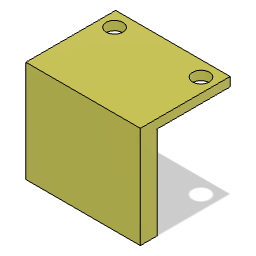
Device 3D Model (Autodesk Fusion 360 archive; units mm, degrees)
design "Accelerometer"
Autodesk Fusion 360 part; units mm, degrees
sketch "Sketch1" plane through (0, 0, 0) normal (0, 1, 0) x (1, 0, 0)
  line L0 (0, 0) -> (20.4, 0)
  line L1 (20.4, 0) -> (20.4, -16)
  line L2 (20.4, -16) -> (0, -16)
  line L3 (0, -16) -> (0, 0)
  dimension "d1" = 20.4
  dimension "d2" = 16
  constraint horizontal L0
  constraint vertical L1
  constraint horizontal L2
  constraint vertical L3
  constraint coincident L0.start L3.end
  measures "d1" distance of L0.start L0.end
  measures "d2" distance of L0.start L2.end
extrude "Extrude1" add sketch "Sketch1" along normal blind 1.6
sketch "Sketch2" plane through (0, 1.6, 0) normal (0, 1, 0) x (-1, 0, 0)
  line L0 (0, 16) -> (-20.4, 16)
  line L1 (-20.4, 16) -> (-20.4, 0)
  line L2 (-20.4, 0) -> (0, 0)
  line L3 (0, 0) -> (0, 16)
  line L4 (0, 1.2) -> (-20.4, 1.2)
  line L5 (0, 16) -> (-1, 16)
  line L6 (-20.4, 16) -> (-19.4, 16)
  line L7 (-1, 16) -> (-1, 0)
  line L8 (-19.4, 16) -> (-19.4, 0)
  circle A0 centre (-2.5, 2.7) radius 1.5
  circle A1 centre (-17.9, 2.7) radius 1.5
  dimension "d5" = 1.2
  dimension "d6" = 1
  dimension "d7" = 1
  dimension "d8" = 1.5
  dimension "d9" = 1.5
  constraint coincident L1 L4.end
  constraint perpendicular L1 L4
  constraint coincident L0.start L3.end
  constraint perpendicular L3 L5
  constraint coincident L0.end L1.start
  constraint perpendicular L1 L6
  constraint coincident L2 L7.end
  constraint perpendicular L2 L7
  constraint coincident L2 L8.end
  constraint perpendicular L2 L8
  constraint tangent L4 A0
  constraint tangent L7 A0
  constraint tangent L4 A1
  constraint tangent L8 A1
  measures "d5" distance of L2.end L4.start
  measures "d6" distance of L0.start L5.end
  measures "d7" distance of L0.end L6.end
  measures "d8" radius of A0
  measures "d9" radius of A1
extrude "Extrude2" cut sketch "Sketch2" against normal blind 15 contours A0 | A1
sketch "Sketch3" plane through (0, 0, 0) normal (0, -1, 0) x (1, 0, 0)
  circle A0 centre (2.5, 2.7) radius 1.5
  circle A1 centre (17.9, 2.7) radius 1.5
  line L0 (20.4, 16) -> (0, 16)
  line L1 (0, 16) -> (0, 0)
  line L2 (0, 0) -> (20.4, 0)
  line L3 (20.4, 0) -> (20.4, 16)
  line L4 (0, 16) -> (20.4, 16)
  line L5 (20.4, 16) -> (20.4, 13)
  line L6 (20.4, 13) -> (0, 13)
  line L7 (0, 13) -> (0, 16)
  dimension "d12" = 3
  constraint horizontal L4
  constraint vertical L5
  constraint horizontal L6
  constraint vertical L7
  constraint coincident L0.end L1.start
  measures "d12" distance of L0.end L6.end
extrude "Extrude3" add sketch "Sketch3" along normal blind 16.5 contours L0 L1 L3 L4 L5 L6 L7

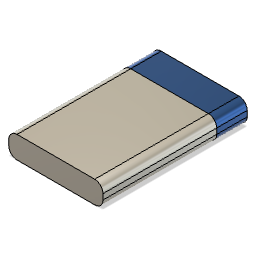
design "Battery"
Autodesk Fusion 360 part; units mm, degrees
sketch "Sketch1" plane through (0, 0, 0) normal (0, 1, 0) x (1, 0, 0)
  line L0 (0, 0) -> (34, 0)
  line L1 (34, 0) -> (34, -52)
  line L2 (34, -52) -> (0, -52)
  line L3 (0, -52) -> (0, 0)
  dimension "d1" = 34
  dimension "d2" = 52
  constraint horizontal L0
  constraint vertical L1
  constraint horizontal L2
  constraint vertical L3
  constraint coincident L0.start L3.end
  measures "d1" distance of L0.start L0.end
  measures "d2" distance of L0.start L2.end
extrude "Extrude1" add sketch "Sketch1" along normal blind 8 makes body 1
fillet "Fillet1" radius 3 4 edges at (34, 8, 26) (34, 0, 26) (0, 8, 26) (0, 0, 26) on bodies 1
ref_plane "WorkPlane1" through (17, 4, 11) normal (0, 0, -1) x (-1, 0, 0)
split "Split1" by plane through (17, 4, 11) normal (0, 0, -1) bodies 1 makes body 2 at (12.3333, 0, 3.6667)
copy_body "Body->Comp1" bodies 1 removing the originals makes body 3 in component "Component"
copy_body "Body->Comp2" bodies 2 removing the originals makes body 4 in component "Component'"
component "Component" placed x (1, 0, 0) y (0, 1, 0) z (0, 0, 1) at (0, 0, 0)
component "Component'" placed x (1, 0, 0) y (0, 1, 0) z (0, 0, 1) at (0, 0, 0)

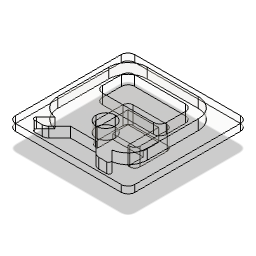
design "Logo"
Autodesk Fusion 360 part; units mm, degrees
sketch "Sketch1" plane through (0, 0, 0) normal (0, 1, 0) x (1, 0, 0)
  line L0 (0, 0) -> (30, 0)
  line L1 (30, 0) -> (30, -30)
  line L2 (30, -30) -> (0, -30)
  line L3 (0, -30) -> (0, 0)
  spline S0 degree 3 poles (5.625, 0) (2.5195, 0) (0, -2.5195) (0, -5.625) knots 0 0 0 0 1 1 1 1
  line L4 (0, -5.625) -> (0, -20.625)
  spline S1 degree 3 poles (0, -20.625) (0, -23.4375) (2.0625, -25.7637) (4.752, -26.1856) knots 0 0 0 0 1 1 1 1
  line L5 (4.752, -26.1856) -> (2.0566, -28.8809)
  spline S2 degree 3 poles (2.0566, -28.8809) (1.6465, -29.2911) (1.9395, -30) (2.5195, -30) knots 0 0 0 0 1 1 1 1
  line L6 (2.5195, -30) -> (4.8457, -30)
  spline S3 degree 3 poles (4.8457, -30) (5.3438, -30) (5.8184, -29.8008) (6.1699, -29.4493) knots 0 0 0 0 1 1 1 1
  line L7 (6.1699, -29.4493) -> (9.375, -26.25)
  line L8 (9.375, -26.25) -> (16.875, -26.25)
  line L9 (16.875, -26.25) -> (20.0742, -29.4493)
  spline S4 degree 3 poles (20.0742, -29.4493) (20.4258, -29.8008) (20.9004, -30) (21.3985, -30) knots 0 0 0 0 1 1 1 1
  line L10 (21.3985, -30) -> (23.7305, -30)
  spline S5 degree 3 poles (23.7305, -30) (24.3164, -30) (24.6094, -29.2911) (24.1934, -28.8809) knots 0 0 0 0 1 1 1 1
  line L11 (24.1934, -28.8809) -> (21.4981, -26.1856)
  spline S6 degree 3 poles (21.4981, -26.1856) (24.1934, -25.7696) (26.25, -23.4375) (26.25, -20.625) knots 0 0 0 0 1 1 1 1
  line L12 (26.25, -20.625) -> (26.25, -5.625)
  spline S7 degree 3 poles (26.25, -5.625) (26.25, -2.5195) (23.7305, 0) (20.625, 0) knots 0 0 0 0 1 1 1 1
  line L13 (20.625, 0) -> (5.625, 0)
  spline S8 degree 3 poles (3.75, -5.625) (3.75, -4.5879) (4.5879, -3.75) (5.625, -3.75) knots 0 0 0 0 1 1 1 1
  line L14 (5.625, -3.75) -> (20.625, -3.75)
  spline S9 degree 3 poles (20.625, -3.75) (21.6621, -3.75) (22.5, -4.5879) (22.5, -5.625) knots 0 0 0 0 1 1 1 1
  line L15 (22.5, -5.625) -> (22.5, -11.25)
  spline S10 degree 3 poles (22.5, -11.25) (22.5, -12.2871) (21.6621, -13.125) (20.625, -13.125) knots 0 0 0 0 1 1 1 1
  line L16 (20.625, -13.125) -> (5.625, -13.125)
  spline S11 degree 3 poles (5.625, -13.125) (4.5879, -13.125) (3.75, -12.2871) (3.75, -11.25) knots 0 0 0 0 1 1 1 1
  line L17 (3.75, -11.25) -> (3.75, -5.625)
  spline S12 degree 3 poles (13.125, -22.5) (11.5723, -22.5) (10.3125, -21.2403) (10.3125, -19.6875) knots 0 0 0 0 1 1 1 1
  spline S13 degree 3 poles (10.3125, -19.6875) (10.3125, -18.1348) (11.5723, -16.875) (13.125, -16.875) knots 0 0 0 0 1 1 1 1
  spline S14 degree 3 poles (13.125, -16.875) (14.6778, -16.875) (15.9375, -18.1348) (15.9375, -19.6875) knots 0 0 0 0 1 1 1 1
  spline S15 degree 3 poles (15.9375, -19.6875) (15.9375, -21.2403) (14.6778, -22.5) (13.125, -22.5) knots 0 0 0 0 1 1 1 1
  dimension "d1" = 30
  dimension "d2" = 30
  constraint horizontal L0
  constraint vertical L1
  constraint horizontal L2
  constraint vertical L3
  constraint coincident L0.start L3.end
  measures "d1" distance of L0.start L0.end
  measures "d2" distance of L0.start L2.end
extrude "Extrude1" add sketch "Sketch1" along normal blind 3 contours L0 L2 L3 S0 L4 S1 L5 S2 L6 S3 L7 L8 L9 S4 L10 S5 L11 S6 L12 S7 L13 makes body 1
sketch "Sketch2" plane through (0, 0, 0) normal (0, -1, 0) x (1, 0, 0)
  spline S0 degree 3 poles (5.625, 13.125) (4.5879, 13.125) (3.75, 12.2871) (3.75, 11.25) knots 0 0 0 0 1 1 1 1
  line L0 (5.625, 13.125) -> (20.625, 13.125)
  spline S1 degree 3 poles (22.5, 11.25) (22.5, 12.2871) (21.6621, 13.125) (20.625, 13.125) knots 0 0 0 0 1 1 1 1
  line L1 (22.5, 11.25) -> (22.5, 5.625)
  spline S2 degree 3 poles (20.625, 3.75) (21.6621, 3.75) (22.5, 4.5879) (22.5, 5.625) knots 0 0 0 0 1 1 1 1
  line L2 (20.625, 3.75) -> (5.625, 3.75)
  spline S3 degree 3 poles (3.75, 5.625) (3.75, 4.5879) (4.5879, 3.75) (5.625, 3.75) knots 0 0 0 0 1 1 1 1
  line L3 (3.75, 5.625) -> (3.75, 11.25)
  spline S4 degree 3 poles (13.125, 16.875) (14.6778, 16.875) (15.9375, 18.1348) (15.9375, 19.6875) knots 0 0 0 0 1 1 1 1
  spline S5 degree 3 poles (10.3125, 19.6875) (10.3125, 18.1348) (11.5723, 16.875) (13.125, 16.875) knots 0 0 0 0 1 1 1 1
  spline S6 degree 3 poles (13.125, 22.5) (11.5723, 22.5) (10.3125, 21.2403) (10.3125, 19.6875) knots 0 0 0 0 1 1 1 1
  spline S7 degree 3 poles (15.9375, 19.6875) (15.9375, 21.2403) (14.6778, 22.5) (13.125, 22.5) knots 0 0 0 0 1 1 1 1
  spline S8 degree 3 poles (23.7383, 30) (24.319, 29.9938) (24.6076, 29.2892) (24.1934, 28.8809) knots 0.004427 0.004427 0.004427 0.004427 1 1 1 1
  line L4 (23.7383, 30) -> (21.386, 30)
  spline S9 degree 3 poles (20.0742, 29.4493) (20.4229, 29.7979) (20.8925, 29.9967) (21.386, 30) knots 0 0 0 0 0.991654 0.991654 0.991654 0.991654
  line L5 (20.0742, 29.4493) -> (16.875, 26.25)
  line L6 (16.875, 26.25) -> (9.375, 26.25)
  line L7 (9.375, 26.25) -> (6.1699, 29.4493)
  spline S10 degree 3 poles (4.8582, 30) (5.3517, 29.9967) (5.8213, 29.7979) (6.1699, 29.4493) knots 0.008346 0.008346 0.008346 0.008346 1 1 1 1
  line L8 (4.8582, 30) -> (2.5118, 30)
  spline S11 degree 3 poles (2.0566, 28.8809) (1.6483, 29.2892) (1.9369, 29.9938) (2.5118, 30) knots 0 0 0 0 0.995573 0.995573 0.995573 0.995573
  line L9 (2.0566, 28.8809) -> (4.752, 26.1856)
  spline S12 degree 3 poles (0, 20.625) (0, 23.4375) (2.0625, 25.7637) (4.752, 26.1856) knots 0 0 0 0 1 1 1 1
  line L10 (0, 20.625) -> (0, 5.625)
  spline S13 degree 3 poles (5.625, 0) (2.5195, 0) (0, 2.5195) (0, 5.625) knots 0 0 0 0 1 1 1 1
  line L11 (5.625, 0) -> (20.625, 0)
  spline S14 degree 3 poles (26.25, 5.625) (26.25, 2.5195) (23.7305, 0) (20.625, 0) knots 0 0 0 0 1 1 1 1
  line L12 (26.25, 5.625) -> (26.25, 20.625)
  spline S15 degree 3 poles (21.4981, 26.1856) (24.1934, 25.7696) (26.25, 23.4375) (26.25, 20.625) knots 0 0 0 0 1 1 1 1
  line L13 (21.4981, 26.1856) -> (24.1934, 28.8809)
  circle A0 centre (13.125, 19.6875) radius 4.1368
extrude "Extrude2" add sketch "Sketch2" along normal blind 1 contours S4 S5 S6 S7 | S8 L4 S9 L5 L6 L7 S10 L8 S11 L9 S12 L10 S13 L11 S14 L12 S15 L13 | A0 bodies 1
sketch "Sketch3" plane through (0, -1, 0) normal (0, -1, 0) x (1, 0, 0)
  spline S0 degree 3 poles (22.5, 5.625) (22.5, 4.5879) (21.6621, 3.75) (20.625, 3.75) knots -1 -1 -1 -1 0 0 0 0
  line L0 (20.625, 3.75) -> (5.625, 3.75)
  spline S1 degree 3 poles (5.625, 3.75) (4.5879, 3.75) (3.75, 4.5879) (3.75, 5.625) knots -1 -1 -1 -1 0 0 0 0
  line L1 (3.75, 5.625) -> (3.75, 11.25)
  spline S2 degree 3 poles (3.75, 11.25) (3.75, 12.2871) (4.5879, 13.125) (5.625, 13.125) knots -1 -1 -1 -1 0 0 0 0
  line L2 (5.625, 13.125) -> (20.625, 13.125)
  spline S3 degree 3 poles (20.625, 13.125) (21.6621, 13.125) (22.5, 12.2871) (22.5, 11.25) knots -1 -1 -1 -1 0 0 0 0
  line L3 (22.5, 11.25) -> (22.5, 5.625)
  line L4 (26.25, 5.625) -> (26.25, 20.625)
  spline S4 degree 3 poles (26.25, 20.625) (26.25, 23.4375) (24.1934, 25.7696) (21.4981, 26.1856) knots -1 -1 -1 -1 0 0 0 0
  line L5 (21.4981, 26.1856) -> (24.1934, 28.8809)
  spline S5 degree 3 poles (24.1934, 28.8809) (24.6076, 29.2892) (24.319, 29.9938) (23.7383, 30) knots -1 -1 -1 -1 -0.004427 -0.004427 -0.004427 -0.004427
  line L6 (23.7383, 30) -> (21.386, 30)
  spline S6 degree 3 poles (21.386, 30) (20.8925, 29.9967) (20.4229, 29.7979) (20.0742, 29.4493) knots -0.991654 -0.991654 -0.991654 -0.991654 0 0 0 0
  line L7 (20.0742, 29.4493) -> (16.875, 26.25)
  line L8 (16.875, 26.25) -> (9.375, 26.25)
  line L9 (9.375, 26.25) -> (6.1699, 29.4493)
  spline S7 degree 3 poles (6.1699, 29.4493) (5.8213, 29.7979) (5.3517, 29.9967) (4.8582, 30) knots -1 -1 -1 -1 -0.008346 -0.008346 -0.008346 -0.008346
  line L10 (4.8582, 30) -> (2.5118, 30)
  spline S8 degree 3 poles (2.5118, 30) (1.9369, 29.9938) (1.6483, 29.2892) (2.0566, 28.8809) knots -0.995573 -0.995573 -0.995573 -0.995573 0 0 0 0
  line L11 (2.0566, 28.8809) -> (4.752, 26.1856)
  spline S9 degree 3 poles (4.752, 26.1856) (2.0625, 25.7637) (0, 23.4375) (0, 20.625) knots -1 -1 -1 -1 0 0 0 0
  line L12 (0, 20.625) -> (0, 5.625)
  spline S10 degree 3 poles (0, 5.625) (0, 2.5195) (2.5195, 0) (5.625, 0) knots -1 -1 -1 -1 0 0 0 0
  line L13 (5.625, 0) -> (20.625, 0)
  spline S11 degree 3 poles (20.625, 0) (23.7305, 0) (26.25, 2.5195) (26.25, 5.625) knots -1 -1 -1 -1 0 0 0 0
  line L14 (23.5046, 3.0171) -> (3, 3.0171)
  line L15 (3, 3.0171) -> (3, 15)
  line L16 (3, 15) -> (23.5046, 15)
  line L17 (23.5046, 15) -> (23.5046, 3.0171)
  constraint horizontal L14
  constraint vertical L15
  constraint horizontal L16
  constraint vertical L17
extrude "Extrude3" add sketch "Sketch3" against normal blind 1 contours S0 L0 S1 L1 S2 L2 S3 L3 bodies 1
sketch "Sketch4" plane through (0, -1, 0) normal (0, -1, 0) x (1, 0, 0)
  line L0 (26.25, 5.625) -> (26.25, 20.625)
  spline S0 degree 3 poles (26.25, 20.625) (26.25, 23.4375) (24.1934, 25.7696) (21.4981, 26.1856) knots -1 -1 -1 -1 0 0 0 0
  line L1 (21.4981, 26.1856) -> (24.1934, 28.8809)
  spline S1 degree 3 poles (24.1934, 28.8809) (24.6076, 29.2892) (24.319, 29.9938) (23.7383, 30) knots -1 -1 -1 -1 -0.004427 -0.004427 -0.004427 -0.004427
  line L2 (23.7383, 30) -> (21.386, 30)
  spline S2 degree 3 poles (21.386, 30) (20.8925, 29.9967) (20.4229, 29.7979) (20.0742, 29.4493) knots -0.991654 -0.991654 -0.991654 -0.991654 0 0 0 0
  line L3 (20.0742, 29.4493) -> (16.875, 26.25)
  line L4 (16.875, 26.25) -> (9.375, 26.25)
  line L5 (9.375, 26.25) -> (6.1699, 29.4493)
  spline S3 degree 3 poles (6.1699, 29.4493) (5.8213, 29.7979) (5.3517, 29.9967) (4.8582, 30) knots -1 -1 -1 -1 -0.008346 -0.008346 -0.008346 -0.008346
  line L6 (4.8582, 30) -> (2.5118, 30)
  spline S4 degree 3 poles (2.5118, 30) (1.9369, 29.9938) (1.6483, 29.2892) (2.0566, 28.8809) knots -0.995573 -0.995573 -0.995573 -0.995573 0 0 0 0
  line L7 (2.0566, 28.8809) -> (4.752, 26.1856)
  spline S5 degree 3 poles (4.752, 26.1856) (2.0625, 25.7637) (0, 23.4375) (0, 20.625) knots -1 -1 -1 -1 0 0 0 0
  line L8 (0, 20.625) -> (0, 5.625)
  spline S6 degree 3 poles (0, 5.625) (0, 2.5195) (2.5195, 0) (5.625, 0) knots -1 -1 -1 -1 0 0 0 0
  line L9 (5.625, 0) -> (20.625, 0)
  spline S7 degree 3 poles (20.625, 0) (23.7305, 0) (26.25, 2.5195) (26.25, 5.625) knots -1 -1 -1 -1 0 0 0 0
  line L10 (10.625, 15.625) -> (15.625, 15.625)
  line L11 (15.625, 15.625) -> (15.625, 10.625)
  line L12 (15.625, 10.625) -> (10.625, 10.625)
  line L13 (10.625, 10.625) -> (10.625, 15.625)
  line L14 (10.625, 15.625) -> (15.625, 10.625) construction
  line L15 (15.625, 15.625) -> (10.625, 10.625) construction
  line L16 (8.625, 17.625) -> (17.625, 17.625)
  line L17 (17.625, 17.625) -> (17.625, 8.625)
  line L18 (17.625, 8.625) -> (8.625, 8.625)
  line L19 (8.625, 8.625) -> (8.625, 17.625)
  line L20 (6.625, 19.625) -> (19.625, 19.625)
  line L21 (19.625, 19.625) -> (19.625, 6.625)
  line L22 (19.625, 6.625) -> (6.625, 6.625)
  line L23 (6.625, 6.625) -> (6.625, 19.625)
  line L24 (17.625, 17.625) -> (19.625, 17.625)
  line L25 (19.625, 17.625) -> (19.625, 6.625)
  line L26 (19.625, 6.625) -> (17.625, 6.625)
  line L27 (17.625, 8.625) -> (17.625, 17.625)
  line L28 (8.625, 17.625) -> (6.625, 17.625)
  line L29 (6.625, 17.625) -> (6.625, 6.625)
  line L30 (6.625, 6.625) -> (8.625, 6.625)
  line L31 (8.625, 8.625) -> (8.625, 17.625)
  dimension "d9" = 5
  dimension "d10" = 5
  dimension "d11" = -2
  dimension "d12" = -4
  constraint horizontal L10
  constraint perpendicular L10 L11
  constraint parallel L10 L12
  constraint parallel L11 L13
  constraint horizontal L24
  constraint vertical L25
  constraint horizontal L26
  constraint vertical L27
  constraint horizontal L28
  constraint vertical L29
  constraint horizontal L30
  constraint vertical L31
  measures "d9" distance of L11.end L12.end
  measures "d10" distance of L10.end L11.end
extrude "Extrude4" add sketch "Sketch4" along normal blind 2.8 contours L17 L18 L19 L21 L22 L23 L24 L25 L26 L27 L28 L29 L30 L31 bodies 1
sketch "Sketch5" plane through (0, -3.8, 0) normal (0, -1, 0) x (1, 0, 0)
  line L0 (17.625, 8.625) -> (8.625, 8.625)
  line L1 (8.625, 8.625) -> (8.625, 17.625)
  line L2 (8.625, 17.625) -> (6.625, 17.625)
  line L3 (6.625, 17.625) -> (6.625, 6.625)
  line L4 (6.625, 6.625) -> (19.625, 6.625)
  line L5 (19.625, 6.625) -> (19.625, 17.625)
  line L6 (19.625, 17.625) -> (17.625, 17.625)
  line L7 (17.625, 17.625) -> (17.625, 8.625)
  line L8 (19.625, 6.625) -> (6.625, 6.625)
  line L9 (6.625, 6.625) -> (6.625, 17.625)
  line L10 (6.625, 17.625) -> (19.625, 17.625)
  line L11 (19.625, 17.625) -> (19.625, 6.625)
  constraint horizontal L8
  constraint vertical L9
  constraint horizontal L10
  constraint vertical L11
  constraint coincident L2.end L3.start
  constraint coincident L4.end L5.start
extrude "Extrude5" add sketch "Sketch5" along normal blind 1.5 bodies 1
fillet "Fillet1" radius 1.5 4 edges at (19.625, -3.15, 6.625) (19.625, -3.15, 17.625) (6.625, -3.15, 17.625) (6.625, -3.15, 6.625) on bodies 1
extrude "Extrude6" cut 1 faces at (11.4584, -5.3, 13.9584) along direction (0, 1, 0) blind 1.5 on bodies 1 bodies 1
extrude "Extrude7" add 1 faces at (7.9584, -3.8, 14.125) along direction (0, -1, 0) blind 1 on bodies 1 bodies 1
sketch "Sketch6" plane through (0, -4.8, 0) normal (0, -1, 0) x (1, 0, 0)
  line L0 (17.625, 17.625) -> (17.625, 8.625)
  line L1 (17.625, 8.625) -> (8.625, 8.625)
  line L2 (8.625, 8.625) -> (8.625, 17.625)
  line L3 (8.625, 17.625) -> (8.125, 17.625)
  arc A0 (8.125, 17.625) -> (6.625, 16.125) centre (8.125, 16.125) ccw
  line L4 (6.625, 16.125) -> (6.625, 8.125)
  arc A1 (6.625, 8.125) -> (8.125, 6.625) centre (8.125, 8.125) ccw
  line L5 (8.125, 6.625) -> (18.125, 6.625)
  arc A2 (18.125, 6.625) -> (19.625, 8.125) centre (18.125, 8.125) ccw
  line L6 (19.625, 8.125) -> (19.625, 16.125)
  arc A3 (19.625, 16.125) -> (18.125, 17.625) centre (18.125, 16.125) ccw
  line L7 (18.125, 17.625) -> (17.625, 17.625)
  line L8 (17.625, 8.625) -> (8.625, 8.625)
  line L9 (8.625, 8.625) -> (8.625, 13.125)
  line L10 (8.625, 13.125) -> (17.625, 13.125)
  line L11 (17.625, 13.125) -> (17.625, 8.625)
  constraint horizontal L8
  constraint vertical L9
  constraint horizontal L10
  constraint vertical L11
  constraint midpoint L2 L9.end
  constraint coincident L0.end L1.start
extrude "Extrude8" add sketch "Sketch6" along normal blind 1 bodies 1
extrude "Extrude9" add 1 faces at (14.625, -5.8, 8.7917) along direction (0, -1, 0) blind 0.5 on bodies 1 bodies 1
sketch "Sketch7" plane through (0, -1, 0) normal (0, -1, 0) x (1, 0, 0)
  line L0 (17.625, 8.625) -> (17.625, 17.625)
  line L1 (17.625, 17.625) -> (18.125, 17.625)
  arc A0 (19.625, 16.125) -> (18.125, 17.625) centre (18.125, 16.125) ccw
  line L2 (19.625, 16.125) -> (19.625, 8.125)
  arc A1 (18.125, 6.625) -> (19.625, 8.125) centre (18.125, 8.125) ccw
  line L3 (18.125, 6.625) -> (8.125, 6.625)
  arc A2 (6.625, 8.125) -> (8.125, 6.625) centre (8.125, 8.125) ccw
  line L4 (6.625, 8.125) -> (6.625, 16.125)
  arc A3 (8.125, 17.625) -> (6.625, 16.125) centre (8.125, 16.125) ccw
  line L5 (8.125, 17.625) -> (8.625, 17.625)
  line L6 (8.625, 17.625) -> (8.625, 8.625)
  line L7 (8.625, 8.625) -> (17.625, 8.625)
  line L8 (26.25, 5.625) -> (26.25, 20.625)
  spline S0 degree 3 poles (26.25, 20.625) (26.25, 23.4375) (24.1934, 25.7696) (21.4981, 26.1856) knots -1 -1 -1 -1 0 0 0 0
  line L9 (21.4981, 26.1856) -> (24.1934, 28.8809)
  spline S1 degree 3 poles (24.1934, 28.8809) (24.6076, 29.2892) (24.319, 29.9938) (23.7383, 30) knots -1 -1 -1 -1 -0.004427 -0.004427 -0.004427 -0.004427
  line L10 (23.7383, 30) -> (21.386, 30)
  spline S2 degree 3 poles (21.386, 30) (20.8925, 29.9967) (20.4229, 29.7979) (20.0742, 29.4493) knots -0.991654 -0.991654 -0.991654 -0.991654 0 0 0 0
  line L11 (20.0742, 29.4493) -> (16.875, 26.25)
  line L12 (16.875, 26.25) -> (9.375, 26.25)
  line L13 (9.375, 26.25) -> (6.1699, 29.4493)
  spline S3 degree 3 poles (6.1699, 29.4493) (5.8213, 29.7979) (5.3517, 29.9967) (4.8582, 30) knots -1 -1 -1 -1 -0.008346 -0.008346 -0.008346 -0.008346
  line L14 (4.8582, 30) -> (2.5118, 30)
  spline S4 degree 3 poles (2.5118, 30) (1.9369, 29.9938) (1.6483, 29.2892) (2.0566, 28.8809) knots -0.995573 -0.995573 -0.995573 -0.995573 0 0 0 0
  line L15 (2.0566, 28.8809) -> (4.752, 26.1856)
  spline S5 degree 3 poles (4.752, 26.1856) (2.0625, 25.7637) (0, 23.4375) (0, 20.625) knots -1 -1 -1 -1 0 0 0 0
  line L16 (0, 20.625) -> (0, 5.625)
  spline S6 degree 3 poles (0, 5.625) (0, 2.5195) (2.5195, 0) (5.625, 0) knots -1 -1 -1 -1 0 0 0 0
  line L17 (5.625, 0) -> (20.625, 0)
  spline S7 degree 3 poles (20.625, 0) (23.7305, 0) (26.25, 2.5195) (26.25, 5.625) knots -1 -1 -1 -1 0 0 0 0
  line L18 (13.125, 0) -> (13.125, 26.25)
  line L19 (26.25, 13.125) -> (0, 13.125)
  line L20 (30.625, 30.625) -> (-4.375, 30.625)
  line L21 (-4.375, 30.625) -> (-4.375, -4.375)
  line L22 (-4.375, -4.375) -> (30.625, -4.375)
  line L23 (30.625, -4.375) -> (30.625, 30.625)
  line L24 (30.625, 30.625) -> (-4.375, -4.375) construction
  line L25 (-4.375, 30.625) -> (30.625, -4.375) construction
  point P0 (13.125, 13.125)
  dimension "d27" = 35
  dimension "d28" = 35
  constraint midpoint L17 L18.start
  constraint midpoint L12 L18.end
  constraint midpoint L8 L19.start
  constraint midpoint L16 L19.end
  constraint horizontal L20
  constraint perpendicular L20 L21
  constraint parallel L20 L22
  constraint parallel L21 L23
  constraint coincident L24 P0
  constraint coincident L25 P0
  constraint midpoint L19 P0
  measures "d27" distance of L21.end L22.end
  measures "d28" distance of L20.end L21.end
extrude "Extrude10" add sketch "Sketch7" against normal blind 1 bodies 1
split "Split1" by plane through (0, -1, 0) normal (0, -1, 0) bodies 1 makes body 2 at (14.625, -6.3, 8.7917)
move_body "Move1" bodies 2 to x (1, 0, 0) y (0, 1, 0) z (0, 0, 1) at (0, -1, 0)
extrude "Extrude11" add 3 faces at (13.125, -1, -2.9167) (13.125, -1, 20.5) (18.2917, -1, 14.125) along direction (0, -1, 0) blind 1 on bodies 1 bodies 1 2
fillet "Fillet2" radius 2 4 edges at (-4.375, -1, 30.625) (30.625, -1, 30.625) (30.625, -1, -4.375) (-4.375, -1, -4.375) on bodies 1
named bodies: "Logo", "Logo (1)"

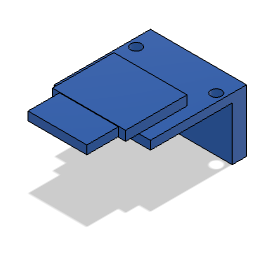
design "SDCard"
Autodesk Fusion 360 part; units mm, degrees
sketch "Sketch1" plane through (0, 0, 0) normal (0, 1, 0) x (1, 0, 0)
  line L0 (0, 0) -> (18, 0)
  line L1 (18, 0) -> (18, -18)
  line L2 (18, -18) -> (0, -18)
  line L3 (0, -18) -> (0, 0)
  dimension "d1" = 18
  dimension "d2" = 18
  constraint horizontal L0
  constraint vertical L1
  constraint horizontal L2
  constraint vertical L3
  constraint coincident L0.start L3.end
  measures "d1" distance of L0.start L0.end
  measures "d2" distance of L0.start L2.end
extrude "Extrude1" add sketch "Sketch1" along normal blind 1.6
sketch "Sketch2" plane through (0, 1.6, 0) normal (0, 1, 0) x (-1, 0, 0)
  line L0 (0, 18) -> (-18, 18)
  line L1 (-18, 18) -> (-18, 0)
  line L2 (-18, 0) -> (0, 0)
  line L3 (0, 0) -> (0, 18)
  line L4 (-9, 3.18) -> (-0.5, 3.18)
  line L5 (-9, 3.18) -> (-17.5, 3.18)
  line L6 (-17.5, 4.4686) -> (-17.5, 3.18)
  line L7 (-17.5, 4.4686) -> (-17.5, 18)
  line L8 (-0.5, 3.18) -> (-0.5, 18)
  circle A0 centre (-3.7436, 6.8938) radius 1
  circle A1 centre (-1.5, 4.18) radius 1
  circle A2 centre (-16.5, 4.18) radius 1
  dimension "d8" = 2
  dimension "d9" = 1
  dimension "d10" = 1
  constraint perpendicular L3 L4
  constraint perpendicular L1 L5
  constraint perpendicular L2 L6
  constraint coincident L0 L7.end
  constraint perpendicular L0 L7
  constraint coincident L0 L8.end
  constraint perpendicular L0 L8
  constraint tangent L4 A1
  constraint tangent L8 A1
  constraint tangent L6 A2
  constraint tangent L5 A2
  measures "d8" diameter of A0
  measures "d9" radius of A1
  measures "d10" radius of A2
extrude "Extrude2" cut sketch "Sketch2" against normal blind 22 contours A1 | A2
sketch "Sketch3" plane through (0, 0, 0) normal (0, -1, 0) x (1, 0, 0)
  circle A0 centre (16.5, 4.18) radius 1
  circle A1 centre (1.5, 4.18) radius 1
  line L0 (18, 18) -> (0, 18)
  line L1 (0, 18) -> (0, 0)
  line L2 (0, 0) -> (18, 0)
  line L3 (18, 0) -> (18, 18)
  line L4 (18, 0) -> (0, 0)
  line L5 (0, 0) -> (0, 2.7)
  line L6 (0, 2.7) -> (18, 2.7)
  line L7 (18, 2.7) -> (18, 0)
  dimension "d13" = 2.7
  constraint horizontal L4
  constraint vertical L5
  constraint horizontal L6
  constraint vertical L7
  constraint coincident L2.end L3.start
  measures "d13" distance of L2.end L6.end
extrude "Extrude3" add sketch "Sketch3" along normal blind 10 contours L1 L2 L3 L4 L5 L6 L7
sketch "Sketch4" plane through (0, 1.6, 0) normal (0, 1, 0) x (-1, 0, 0)
  circle A0 centre (-16.5, 4.18) radius 1
  circle A1 centre (-1.5, 4.18) radius 1
  line L0 (0, 18) -> (-18, 18)
  line L1 (-18, 18) -> (-18, 0)
  line L2 (-18, 0) -> (0, 0)
  line L3 (0, 0) -> (0, 18)
  line L4 (18.2773, 7.6692) -> (4.5773, 7.6692)
  line L5 (4.5773, 7.6692) -> (4.5773, 19.1692)
  line L6 (4.5773, 19.1692) -> (18.2773, 19.1692)
  line L7 (18.2773, 19.1692) -> (18.2773, 7.6692)
  line L8 (-1.586, 18) -> (-1.586, 9)
  line L9 (-9, 18) -> (-9, 9)
  line L10 (-9, 9) -> (-2.15, 9)
  line L11 (-9, 9) -> (-15.85, 9)
  line L12 (-2.15, 9) -> (-2.15, 20.5)
  line L13 (-2.15, 20.5) -> (-15.85, 20.5)
  line L14 (-15.85, 20.5) -> (-15.85, 9)
  dimension "d16" = 13.7
  dimension "d17" = 11.5
  dimension "d18" = 6.85
  dimension "d19" = 6.85
  dimension "d20" = 11.5
  constraint horizontal L4
  constraint vertical L5
  constraint horizontal L6
  constraint vertical L7
  constraint coincident L0 L8.start
  constraint perpendicular L0 L8
  constraint midpoint L0 L9.start
  constraint perpendicular L0 L9
  constraint perpendicular L8 L10
  constraint perpendicular L9 L11
  constraint perpendicular L0 L12
  constraint perpendicular L12 L13
  constraint perpendicular L11 L14
  measures "d16" distance of L4.start L4.end
  measures "d17" distance of L4.start L6.end
  measures "d18" distance of L9.end L10.end
  measures "d19" distance of L9.end L11.end
  measures "d20" distance of L10.end L12.end
extrude "Extrude4" add sketch "Sketch4" along normal blind 1.8 contours L0 L9 L10 L12 | L0 L12 L13 L14 | L0 L9 L11 L14
sketch "Sketch5" plane through (0, 0, 20.5) normal (0, 0, 1) x (1, 0, 0)
  line L0 (2.15, 1.6) -> (15.85, 1.6)
  line L1 (15.85, 1.6) -> (15.85, 3.4)
  line L2 (15.85, 3.4) -> (2.15, 3.4)
  line L3 (2.15, 3.4) -> (2.15, 1.6)
  line L4 (3.5, 3.3) -> (14.5, 3.3)
  line L5 (14.5, 3.3) -> (14.5, 1.7)
  line L6 (14.5, 1.7) -> (3.5, 1.7)
  line L7 (3.5, 1.7) -> (3.5, 3.3)
  line L8 (3.5, 3.3) -> (14.5, 1.7) construction
  line L9 (14.5, 3.3) -> (3.5, 1.7) construction
  point P0 (9, 2.5)
  dimension "d23" = 11
  dimension "d24" = 1.6
  constraint horizontal L4
  constraint perpendicular L4 L5
  constraint parallel L4 L6
  constraint parallel L5 L7
  constraint coincident L8 P0
  constraint coincident L9 P0
  measures "d23" distance of L5.end L6.end
  measures "d24" distance of L4.end L5.end
extrude "Extrude5" add sketch "Sketch5" along normal blind 5.9 contours L4 L5 L6 L7
equation "d18 = ( 13.7 / 2 ) * 1 mm"
